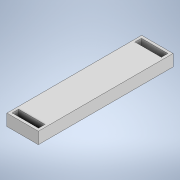
# Autodesk Inventor part: Leg
Saved by Autodesk Inventor 2021 (Build 250183000, 183)
## iProperties
Created: 2024-05-05
Part Number: Leg
Material: Generic
Document SubType Name: Modeling
Designer: brybr
Density: 1 g/cm^3
Appearance: Default
Author: brybr
Autodesk Inventor part; units mm, degrees
ref_plane "YZ Plane" through (0, 0, 0) normal (1, 0, 0) x (0, 1, 0)
ref_plane "XZ Plane" through (0, 0, 0) normal (0, 1, 0) x (-1, 0, 0)
ref_plane "XY Plane" through (0, 0, 0) normal (0, 0, 1) x (1, 0, 0)
sketch "Sketch1" plane through (0, 0, 0) normal (0, 0, 1) x (1, 0, 0)
  line L0 (-17.5, 6.5) -> (17.5, 6.5)
  line L1 (17.5, 6.5) -> (17.5, -6.5)
  line L2 (17.5, -6.5) -> (-17.5, -6.5)
  line L3 (-17.5, -6.5) -> (-17.5, 6.5)
  line L4 (-17.5, 6.5) -> (17.5, -6.5) construction
  line L5 (17.5, 6.5) -> (-17.5, -6.5) construction
  line L6 (-17.5, 6.5) -> (17.5, 6.5) construction
  point P0 (0, 0)
  dimension "d0" = 35
  dimension "d1" = 0
  dimension "d2" = 13
  constraints: 14 end point, 2 horizontal, 2 midpoint, 2 parallel, 1 collinear, 1 perpendicular
  measures "d0" distance of L0.start L0.end
  measures "d1" distance between parallel lines of L0 L6
  measures "d2" distance of L0.end L1.end
extrude "Extrusion1" add sketch "Sketch1" along normal blind 150
sketch "Sketch2" plane through (-17.5, 6.5, 0) normal (0, 1, 0) x (1, 0, 0)
  line L0 (2.8, -10.2) -> (32.2, -10.2)
  line L1 (32.2, -10.2) -> (32.2, -3)
  line L2 (32.2, -3) -> (2.8, -3)
  line L3 (2.8, -3) -> (2.8, -10.2)
  line L4 (2.8, -10.2) -> (32.2, -3) construction
  line L5 (32.2, -10.2) -> (2.8, -3) construction
  line L6 (2.8, -10.2) -> (32.2, -10.2) construction
  line L7 (2.8, -6.6) -> (0, -6.6)
  line L8 (0, 0) -> (0, -150) projected
  line L9 (35, 0) -> (35, -150) projected
  line L10 (35, -6.6) -> (32.2, -6.6)
  line L11 (35, 0) -> (0, 0) projected
  line L12 (2.8, -147) -> (32.2, -147)
  line L13 (32.2, -147) -> (32.2, -139.8)
  line L14 (32.2, -139.8) -> (2.8, -139.8)
  line L15 (2.8, -139.8) -> (2.8, -147)
  line L16 (2.8, -147) -> (32.2, -139.8) construction
  line L17 (32.2, -147) -> (2.8, -139.8) construction
  line L18 (2.8, -147) -> (32.2, -147) construction
  line L19 (2.8, -143.4) -> (0, -143.4)
  line L20 (35, -143.4) -> (32.2, -143.4)
  line L21 (35, -150) -> (0, -150) projected
  point P0 (17.5, 0)
  point P1 (17.5, -6.6)
  point P2 (17.5, -143.4)
  dimension "d6" = 29.4
  dimension "d8" = 7.2
  dimension "d9" = 3
  dimension "d12" = 29.4
  dimension "d13" = 0
  dimension "d14" = 7.2
  dimension "d15" = 3
  constraints: 36 end point, 8 midpoint, 6 horizontal, 6 point on line, 4 collinear, 4 parallel, 2 perpendicular
  measures "d6" distance of L0.start L0.end
  measures "d8" distance of L1.end L0.end
  measures "d9" distance between parallel lines of L11 L2
  measures "d12" distance of L12.start L12.end
  measures "d13" distance between parallel lines of L12 L18
  measures "d14" distance of L13.end L12.end
  measures "d15" distance between parallel lines of L21 L12
extrude "Extrusion2" cut sketch "Sketch2" against normal through all contours L3 L2 L1 L0 | L15 L14 L13 L12
body "Solid1"
